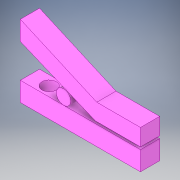
# Autodesk Inventor part: pince a linge
Saved by Autodesk Inventor 2019 (Build 230136000, 136)
## iProperties
Created: 2020-02-15
Part Number: pince a linge
Material: Generic
Document SubType Name: Modeling
Designer: franc
Density: 1 g/cm^3
Appearance: Default
Author: franc
Autodesk Inventor part; units mm, degrees
ref_plane "YZ Plane" through (0, 0, 0) normal (1, 0, 0) x (0, 1, 0)
ref_plane "XZ Plane" through (0, 0, 0) normal (0, 1, 0) x (-1, 0, 0)
ref_plane "XY Plane" through (0, 0, 0) normal (0, 0, 1) x (1, 0, 0)
sketch "Esquisse1" plane through (0, 0, 0) normal (0, 1, 0) x (-1, 0, 0)
  line L0 (2.5091, 2.6545) -> (-22.4909, 2.6545)
  line L1 (-22.4909, 2.6545) -> (-22.4909, -1.3455)
  line L2 (-22.4909, -1.3455) -> (2.5091, -1.3455)
  line L3 (2.5091, -1.3455) -> (2.5091, 2.6545)
  point P0 (0, 0)
  dimension "d0" = 4
  dimension "d1" = 25
  constraints: 8 end point, 2 parallel, 1 horizontal, 1 perpendicular
  measures "d0" distance of L2.end L0.start
  measures "d1" distance of L1.end L2.end
extrude "Extrusion1" add sketch "Esquisse1" along normal blind 4
sketch "Esquisse3" plane through (22.4909, 0, -1.3455) normal (0, 0, -1) x (-1, 0, 0)
  circle A0 centre (16, 5.5) radius 1.5
  line L0 (0, 4) -> (25, 4) projected
  line L1 (25, 0) -> (25, 4) projected
  point P0 (22.4909, 0)
  dimension "d4" = 3
  dimension "d5" = 1.5
  dimension "d6" = 9
  constraints: 1 centre point
  measures "d4" diameter of A0
  measures "d5" distance from line of L0 A0.centre
  measures "d6" distance from line of L1 A0.centre
extrude "Extrusion2" add sketch "Esquisse3" against normal blind 4
sketch "Esquisse4" plane through (22.4909, 0, -1.3455) normal (0, 0, -1) x (-1, 0, 0)
  line L0 (0, 4) -> (16, 4) projected
  line L1 (25, 11) -> (9.4076, 4.5)
  line L2 (25, 0) -> (25, 4) projected
  line L3 (16, 4) -> (25, 4) projected
  line L4 (25, 11) -> (25, 15)
  line L5 (25, 15) -> (9.0943, 8)
  line L6 (9.0943, 8) -> (0, 8)
  line L7 (0, 8) -> (0, 4)
  line L8 (9.4076, 4.5) -> (0, 4.5)
  point P0 (22.4909, 0)
  point P1 (9.0943, 4)
  dimension "d9" = 0
  dimension "d10" = 7
  dimension "d11" = 4
  dimension "d12" = 4
  dimension "d15" = 0.5
  constraints: 12 end point, 3 perpendicular, 2 point on line, 1 vertical
  measures "d9" distance from line of L2 L1.start
  measures "d10" distance from line of L3 L1.start
  measures "d11" distance of L1.start L4.end
  measures "d12" distance of L6.end L0.start
  measures "d15" distance between parallel lines of L0 L8
extrude "Extrusion3" add sketch "Esquisse4" against normal blind 4
sketch "Esquisse6" plane through (0, 0, 0) normal (0, -1, 0) x (1, 0, 0)
  circle A0 centre (1.4909, 0.6545) radius 1.5
  line L0 (22.4909, -1.3455) -> (-2.5091, -1.3455) projected
  line L1 (-2.5091, -1.3455) -> (-2.5091, 2.6545) projected
  point P0 (0, 0)
  dimension "d16" = 3
  dimension "d17" = 2
  dimension "d18" = 4
  constraints: 1 centre point
  measures "d16" diameter of A0
  measures "d17" distance from line of L0 A0.centre
  measures "d18" distance from line of L1 A0.centre
extrude "Extrusion4" cut sketch "Esquisse6" against normal up to next
